Autodesk Fusion 360 part; units mm, degrees
note: some values were not read from the file. Set by a fixed rule: the direction of a hole.
(part 6 of 6)
  line L797 (76.9709, -66.8937) -> (77.185, -66.7888)
  line L798 (77.185, -66.7888) -> (77.3791, -66.6503)
  line L799 (77.3791, -66.6503) -> (77.548, -66.482)
  line L800 (77.548, -66.482) -> (77.6872, -66.2884)
  line L801 (77.6872, -66.2884) -> (77.7928, -66.0746)
  line L802 (77.7928, -66.0746) -> (77.8621, -65.8465)
  line L803 (77.8621, -65.8465) -> (77.8932, -65.6101)
  line L804 (77.8932, -65.6101) -> (77.895, -65.539)
  line L805 (77.895, -65.539) -> (77.8754, -65.3014)
  line L806 (77.8754, -65.3014) -> (77.8173, -65.0701)
  line L807 (77.8173, -65.0701) -> (77.7223, -64.8515)
  line L808 (77.7223, -64.8515) -> (77.5928, -64.6513)
  line L809 (77.5928, -64.6513) -> (77.4323, -64.4749)
  line L810 (77.4323, -64.4749) -> (77.2452, -64.3271)
  line L811 (77.2452, -64.3271) -> (77.0364, -64.2119)
  line L812 (77.0364, -64.2119) -> (76.8117, -64.1323)
  line L813 (76.8117, -64.1323) -> (76.5769, -64.0905)
  line L814 (76.5769, -64.0905) -> (76.3385, -64.0876)
  line L815 (76.3385, -64.0876) -> (76.1028, -64.1236)
  line L816 (76.1028, -64.1236) -> (75.8762, -64.1977)
  line L817 (75.8762, -64.1977) -> (75.6647, -64.3078)
  line L818 (75.6647, -64.3078) -> (75.474, -64.451)
  line L819 (75.474, -64.451) -> (75.3093, -64.6234)
  line L820 (75.3093, -64.6234) -> (75.1749, -64.8203)
  line L821 (75.1749, -64.8203) -> (75.0745, -65.0366)
  line L822 (75.0745, -65.0366) -> (75.0108, -65.2664)
  line L823 (75.0108, -65.2664) -> (74.9855, -65.5035)
  line L824 (74.9855, -65.5035) -> (74.9992, -65.7415)
  line L825 (74.9992, -65.7415) -> (75.0516, -65.9741)
  line L826 (110.529, -65.06) -> (110.622, -64.8353)
  line L827 (110.622, -64.8353) -> (110.749, -64.6279)
  line L828 (110.749, -64.6279) -> (110.907, -64.443)
  line L829 (110.907, -64.443) -> (111.092, -64.285)
  line L830 (111.092, -64.285) -> (111.299, -64.1579)
  line L831 (111.299, -64.1579) -> (111.524, -64.0649)
  line L832 (111.524, -64.0649) -> (111.761, -64.0081)
  line L833 (111.761, -64.0081) -> (112.003, -63.989)
  line L834 (112.003, -63.989) -> (112.245, -64.0081)
  line L835 (112.245, -64.0081) -> (112.482, -64.0649)
  line L836 (112.482, -64.0649) -> (112.707, -64.1579)
  line L837 (112.707, -64.1579) -> (112.914, -64.285)
  line L838 (112.914, -64.285) -> (113.099, -64.443)
  line L839 (113.099, -64.443) -> (113.257, -64.6279)
  line L840 (113.257, -64.6279) -> (113.384, -64.8353)
  line L841 (113.384, -64.8353) -> (113.477, -65.06)
  line L842 (113.477, -65.06) -> (113.534, -65.2965)
  line L843 (113.534, -65.2965) -> (113.553, -65.539)
  line L844 (113.553, -65.539) -> (113.534, -65.7815)
  line L845 (113.534, -65.7815) -> (113.477, -66.018)
  line L846 (113.477, -66.018) -> (113.384, -66.2427)
  line L847 (113.384, -66.2427) -> (113.257, -66.4501)
  line L848 (113.257, -66.4501) -> (113.099, -66.635)
  line L849 (113.099, -66.635) -> (112.914, -66.793)
  line L850 (112.914, -66.793) -> (112.707, -66.9201)
  line L851 (112.707, -66.9201) -> (112.482, -67.0131)
  line L852 (112.482, -67.0131) -> (112.245, -67.0699)
  line L853 (112.245, -67.0699) -> (112.003, -67.089)
  line L854 (112.003, -67.089) -> (111.761, -67.0699)
  line L855 (111.761, -67.0699) -> (111.524, -67.0131)
  line L856 (111.524, -67.0131) -> (111.299, -66.9201)
  line L857 (111.299, -66.9201) -> (111.092, -66.793)
  line L858 (111.092, -66.793) -> (110.907, -66.635)
  line L859 (110.907, -66.635) -> (110.749, -66.4501)
  line L860 (110.749, -66.4501) -> (110.622, -66.2427)
  line L861 (110.622, -66.2427) -> (110.529, -66.018)
  line L862 (110.529, -66.018) -> (110.472, -65.7815)
  line L863 (110.472, -65.7815) -> (110.453, -65.539)
  line L864 (110.453, -65.539) -> (110.456, -65.5035)
  line L865 (110.456, -65.5035) -> (110.472, -65.2965)
  line L866 (110.472, -65.2965) -> (110.529, -65.06)
  line L867 (110.615, -65.9741) -> (110.704, -66.195)
  line L868 (110.704, -66.195) -> (110.829, -66.3983)
  line L869 (110.829, -66.3983) -> (110.985, -66.5785)
  line L870 (110.985, -66.5785) -> (111.168, -66.7308)
  line L871 (111.168, -66.7308) -> (111.374, -66.8511)
  line L872 (111.374, -66.8511) -> (111.597, -66.9362)
  line L873 (111.597, -66.9362) -> (111.831, -66.9837)
  line L874 (111.831, -66.9837) -> (112.069, -66.9925)
  line L875 (112.069, -66.9925) -> (112.306, -66.9622)
  line L876 (112.306, -66.9622) -> (112.534, -66.8937)
  line L877 (112.534, -66.8937) -> (112.748, -66.7888)
  line L878 (112.748, -66.7888) -> (112.942, -66.6503)
  line L879 (112.942, -66.6503) -> (113.111, -66.482)
  line L880 (113.111, -66.482) -> (113.25, -66.2884)
  line L881 (113.25, -66.2884) -> (113.356, -66.0746)
  line L882 (113.356, -66.0746) -> (113.425, -65.8465)
  line L883 (113.425, -65.8465) -> (113.456, -65.6101)
  line L884 (113.456, -65.6101) -> (113.458, -65.539)
  line L885 (113.458, -65.539) -> (113.438, -65.3014)
  line L886 (113.438, -65.3014) -> (113.38, -65.0701)
  line L887 (113.38, -65.0701) -> (113.285, -64.8515)
  line L888 (113.285, -64.8515) -> (113.156, -64.6513)
  line L889 (113.156, -64.6513) -> (112.995, -64.4749)
  line L890 (112.995, -64.4749) -> (112.808, -64.3271)
  line L891 (112.808, -64.3271) -> (112.599, -64.2119)
  line L892 (112.599, -64.2119) -> (112.375, -64.1323)
  line L893 (112.375, -64.1323) -> (112.14, -64.0905)
  line L894 (112.14, -64.0905) -> (111.902, -64.0876)
  line L895 (111.902, -64.0876) -> (111.666, -64.1236)
  line L896 (111.666, -64.1236) -> (111.439, -64.1977)
  line L897 (111.439, -64.1977) -> (111.228, -64.3078)
  line L898 (111.228, -64.3078) -> (111.037, -64.451)
  line L899 (111.037, -64.451) -> (110.872, -64.6234)
  line L900 (110.872, -64.6234) -> (110.738, -64.8203)
  line L901 (110.738, -64.8203) -> (110.638, -65.0366)
  line L902 (110.638, -65.0366) -> (110.574, -65.2664)
  line L903 (110.574, -65.2664) -> (110.548, -65.5035)
  line L904 (110.548, -65.5035) -> (110.562, -65.7415)
  line L905 (110.562, -65.7415) -> (110.615, -65.9741)
  line L906 (39.4089, -65.06) -> (39.5019, -64.8353)
  line L907 (39.5019, -64.8353) -> (39.629, -64.6279)
  line L908 (39.629, -64.6279) -> (39.787, -64.443)
  line L909 (39.787, -64.443) -> (39.9719, -64.285)
  line L910 (39.9719, -64.285) -> (40.1793, -64.1579)
  line L911 (40.1793, -64.1579) -> (40.404, -64.0649)
  line L912 (40.404, -64.0649) -> (40.6405, -64.0081)
  line L913 (40.6405, -64.0081) -> (40.883, -63.989)
  line L914 (40.883, -63.989) -> (41.1255, -64.0081)
  line L915 (41.1255, -64.0081) -> (41.362, -64.0649)
  line L916 (41.362, -64.0649) -> (41.5867, -64.1579)
  line L917 (41.5867, -64.1579) -> (41.7941, -64.285)
  line L918 (41.7941, -64.285) -> (41.979, -64.443)
  line L919 (41.979, -64.443) -> (42.137, -64.6279)
  line L920 (42.137, -64.6279) -> (42.2641, -64.8353)
  line L921 (42.2641, -64.8353) -> (42.3571, -65.06)
  line L922 (42.3571, -65.06) -> (42.4139, -65.2965)
  line L923 (42.4139, -65.2965) -> (42.433, -65.539)
  line L924 (42.433, -65.539) -> (42.4139, -65.7815)
  line L925 (42.4139, -65.7815) -> (42.3571, -66.018)
  line L926 (42.3571, -66.018) -> (42.2641, -66.2427)
  line L927 (42.2641, -66.2427) -> (42.137, -66.4501)
  line L928 (42.137, -66.4501) -> (41.979, -66.635)
  line L929 (41.979, -66.635) -> (41.7941, -66.793)
  line L930 (41.7941, -66.793) -> (41.5867, -66.9201)
  line L931 (41.5867, -66.9201) -> (41.362, -67.0131)
  line L932 (41.362, -67.0131) -> (41.1255, -67.0699)
  line L933 (41.1255, -67.0699) -> (40.883, -67.089)
  line L934 (40.883, -67.089) -> (40.6405, -67.0699)
  line L935 (40.6405, -67.0699) -> (40.404, -67.0131)
  line L936 (40.404, -67.0131) -> (40.1793, -66.9201)
  line L937 (40.1793, -66.9201) -> (39.9719, -66.793)
  line L938 (39.9719, -66.793) -> (39.787, -66.635)
  line L939 (39.787, -66.635) -> (39.629, -66.4501)
  line L940 (39.629, -66.4501) -> (39.5019, -66.2427)
  line L941 (39.5019, -66.2427) -> (39.4089, -66.018)
  line L942 (39.4089, -66.018) -> (39.3521, -65.7815)
  line L943 (39.3521, -65.7815) -> (39.333, -65.539)
  line L944 (39.333, -65.539) -> (39.3358, -65.5035)
  line L945 (39.3358, -65.5035) -> (39.3521, -65.2965)
  line L946 (39.3521, -65.2965) -> (39.4089, -65.06)
  line L947 (39.4946, -65.9741) -> (39.5843, -66.195)
  line L948 (39.5843, -66.195) -> (39.7089, -66.3983)
  line L949 (39.7089, -66.3983) -> (39.865, -66.5785)
  line L950 (39.865, -66.5785) -> (40.0485, -66.7308)
  line L951 (40.0485, -66.7308) -> (40.2543, -66.8511)
  line L952 (40.2543, -66.8511) -> (40.4771, -66.9362)
  line L953 (40.4771, -66.9362) -> (40.7107, -66.9837)
  line L954 (40.7107, -66.9837) -> (40.949, -66.9925)
  line L955 (40.949, -66.9925) -> (41.1855, -66.9622)
  line L956 (41.1855, -66.9622) -> (41.4139, -66.8937)
  line L957 (41.4139, -66.8937) -> (41.628, -66.7888)
  line L958 (41.628, -66.7888) -> (41.8221, -66.6503)
  line L959 (41.8221, -66.6503) -> (41.991, -66.482)
  line L960 (41.991, -66.482) -> (42.1302, -66.2884)
  line L961 (42.1302, -66.2884) -> (42.2358, -66.0746)
  line L962 (42.2358, -66.0746) -> (42.3051, -65.8465)
  line L963 (42.3051, -65.8465) -> (42.3362, -65.6101)
  line L964 (42.3362, -65.6101) -> (42.338, -65.539)
  line L965 (42.338, -65.539) -> (42.3184, -65.3014)
  line L966 (42.3184, -65.3014) -> (42.2603, -65.0701)
  line L967 (42.2603, -65.0701) -> (42.1653, -64.8515)
  line L968 (42.1653, -64.8515) -> (42.0358, -64.6513)
  line L969 (42.0358, -64.6513) -> (41.8753, -64.4749)
  line L970 (41.8753, -64.4749) -> (41.6882, -64.3271)
  line L971 (41.6882, -64.3271) -> (41.4794, -64.2119)
  line L972 (41.4794, -64.2119) -> (41.2547, -64.1323)
  line L973 (41.2547, -64.1323) -> (41.0199, -64.0905)
  line L974 (41.0199, -64.0905) -> (40.7815, -64.0876)
  line L975 (40.7815, -64.0876) -> (40.5458, -64.1236)
  line L976 (40.5458, -64.1236) -> (40.3192, -64.1977)
  line L977 (40.3192, -64.1977) -> (40.1077, -64.3078)
  line L978 (40.1077, -64.3078) -> (39.917, -64.451)
  line L979 (39.917, -64.451) -> (39.7523, -64.6234)
  line L980 (39.7523, -64.6234) -> (39.6179, -64.8203)
  line L981 (39.6179, -64.8203) -> (39.5175, -65.0366)
  line L982 (39.5175, -65.0366) -> (39.4538, -65.2664)
  line L983 (39.4538, -65.2664) -> (39.4285, -65.5035)
  line L984 (39.4285, -65.5035) -> (39.4422, -65.7415)
  line L985 (39.4422, -65.7415) -> (39.4946, -65.9741)
extrude "Extrude1" add sketch "SOLDERBREAD02_DXF_Outline_in_MilliMeters" along normal blind 2.54 contours L411 L412 L413 L414 L415 L416 L417 L418 L419 L420 L421 L422 L423 L424 L425 L426 L427 L428 L429 L430 L433 L434 L435 L436 L437 L440 L443 L444 L445 L446 L447 L450 L451 L452 L453 L454 L455 L456 L457 L458 L459 L460 L461 L462 L463 L464 L465 L466 L467 L468 L469 L470 L471 L472 L473 L474 L475 L476 L477 L478 L479 L480 L481 L482 L483 L484 L485 L486 L487 L488 L489 L490 L491 L492 L493 L494 L495 L496 L497 L498 L499 L500 L501 L502 L503 L504 L505 L506 L507 L508 L509 L510 L511 L512 L513 L514 L515 L516 L517 L518 L519 L520 L521 L523 L524 L525 L526 L527 L528 L529 L532 L533 L534 L535 L536 L537 L538 L539 L540 L541 L542 L543 L544 L545 L546 L547 L548 L549 L550 L551 L552 L553 L554 L555 L556 L557 L558 L559 L560 L561 L562 L563 L564 L565 L566 L567 L568 L569 L570 L571 L572 L573 L574 L575 L576 L577 L578 L579 L580 L581 L582 L583 L584 L585 L586 L587 L588 L589 L590 L591 L592 L593 L594 L595 L596 L599 L600 L601 L602 L603 L604 L605 L608 L609 L610 L611 L612 L616 L617 L618 L619 L620 L621 L622 L623 L624 L625 L626 L627 L628 L629 L630 L631 L632 L633 L634 L635 L636 L637 L638 L639 L640 L641 L642 L643 L644 L645 L646 L647 L648 L649 L650 L651 L652 L653 L654 L655 L656 L657 L658 L659 L660 L661 L662 L663 L664 L665 L666 L667 L668 L669 L670 L671 L672 L673 L674 L675 L676 L677 L678 L679 L680 L681 L682 L684 L685 L686 L687 L688 L689 L690 L691 L692 L693 L694 L695 L696 L697 L700 L701 L702 L703 L704 L705 L706 L707 L708 L709 L710 L711 L712 L713 L714 L715 L716 L717 L718 L719 L720 L721 L722 L723 L724 L725 L726 L727 L728 L729 L730 L731 L732 L733 L734 L735 L736 L737 L738 L739 L740 L741 L742 L743 L744 L745
